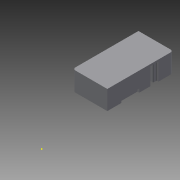
# Autodesk Inventor part: Positive CAp
Saved by Autodesk Inventor 2015 (Build 190159000, 159)
## iProperties
Created: 2015-01-23
Part Number: Positive CAp
Material: Generic
Document SubType Name: Modeling
Designer: pltwe4
Density: 1 g/cm^3
Appearance: Default
Author: pltwe4
Autodesk Inventor part; units mm, degrees
ref_plane "YZ Plane" through (0, 0, 0) normal (1, 0, 0) x (0, 1, 0)
ref_plane "XZ Plane" through (0, 0, 0) normal (0, 1, 0) x (-1, 0, 0)
ref_plane "XY Plane" through (0, 0, 0) normal (0, 0, 1) x (1, 0, 0)
sketch "Sketch1" plane through (0, 0, 0) normal (0, 1, 0) x (-1, 0, 0)
  line L0 (0, 0) -> (24.5364, 0)
  line L1 (24.5364, 0) -> (24.5364, -46.5582)
  line L2 (24.5364, -46.5582) -> (0, -46.5582)
  line L3 (0, -46.5582) -> (0, 0)
  dimension "d0" = 46.5582
  dimension "d1" = 24.5364
  constraints: 8 end point, 2 parallel, 1 horizontal, 1 perpendicular
  measures "d0" distance of L0.end L1.end
  measures "d1" distance of L1.end L2.end
extrude "Extrusion1" add sketch "Sketch1" along normal blind 13.5382
sketch "Sketch2" plane through (0, 0, 0) normal (0, -1, 0) x (1, 0, 0)
  point P0 (0, 0)
fillet "Fillet1" radius 1.905 1 edges at (-24.5364, 6.7691, -46.5582)
fillet "Fillet2" radius 1.905 1 edges at (0, 6.7691, 0)
sketch "Sketch3" plane through (0, 0, 0) normal (0, -1, 0) x (1, 0, 0)
  line L0 (-1.905, 0) -> (-24.5364, 0) projected
  arc A0 (0, -1.905) -> (-1.905, 0) centre (-1.905, -1.905) ccw projected
  line L1 (0, -46.5582) -> (0, -1.905) projected
  line L2 (-22.6314, -46.5582) -> (0, -46.5582) projected
  arc A1 (-24.5364, -44.6532) -> (-22.6314, -46.5582) centre (-22.6314, -44.6532) ccw projected
  line L3 (-24.5364, 0) -> (-24.5364, -44.6532) projected
  line L4 (-2.54, -2.54) -> (-21.9964, -2.54)
  line L5 (-21.9964, -44.0182) -> (-2.54, -44.0182)
  line L6 (0, -12.9032) -> (-5.08, -12.9032)
  line L7 (-5.08, -16.0782) -> (0, -16.0782)
  line L8 (-2.54, -44.0182) -> (-2.54, -18.6182)
  line L9 (-2.54, -10.3632) -> (-2.54, -2.54)
  line L10 (-5.08, -12.9032) -> (-5.08, -10.3632)
  line L11 (-5.08, -10.3632) -> (-2.54, -10.3632)
  line L12 (-5.08, -16.0782) -> (-5.08, -18.6182)
  line L13 (-5.08, -18.6182) -> (-2.54, -18.6182)
  line L14 (-21.9964, -10.3632) -> (-18.4404, -10.3632)
  line L15 (-18.4404, -10.3632) -> (-18.4404, -18.6182)
  line L16 (-18.4404, -18.6182) -> (-21.9964, -18.6182)
  line L17 (-21.9964, -2.54) -> (-21.9964, -10.3632)
  line L18 (-21.9964, -18.6182) -> (-21.9964, -44.0182)
  line L19 (0, -14.4907) -> (-5.2569, -14.4907) construction
  line L20 (-5.08, -11.6332) -> (-18.4404, -11.6332)
  line L21 (-5.08, -17.3482) -> (-18.4404, -17.3482)
  point P0 (0, 0)
  dimension "d7" = 2.54
  dimension "d9" = 2.54
  dimension "d11" = 3.175
  dimension "d13" = 5.08
  dimension "d14" = 2.54
  dimension "d15" = 2.54
  dimension "d16" = 2.54
  dimension "d17" = 2.54
  dimension "d20" = 2.54
  dimension "d21" = 6.096
  dimension "d22" = 2.54
  dimension "d37" = 32.0675
  constraints: 36 end point, 9 perpendicular, 7 parallel, 5 point on line, 4 horizontal, 2 collinear, 2 midpoint, 2 vertical, 1 other
  measures "d7" distance between parallel lines of L0 L4
  measures "d9" distance between parallel lines of L2 L5
  measures "d11" distance between parallel lines of L6 L7
  measures "d13" distance between parallel lines of L1 L10
  measures "d14" distance of L7.start L12.end
  measures "d15" distance of L6.end L10.end
  measures "d16" distance between parallel lines of L1 L8
  measures "d17" distance between parallel lines of L1 L9
  measures "d20" distance between parallel lines of L3 L18
  measures "d21" distance between parallel lines of L3 L15
  measures "d22" distance between parallel lines of L3 L17
  measures "d37" distance between parallel lines of L2 L19
extrude "Extrusion2" cut sketch "Sketch3" against normal blind 12.2682 contours L1 L7 L12 L21 L15 L20 L10 L6 | L20 L15 L14 L17 L4 L9 L11 L10 | L12 L13 L8 L5 L18 L16 L15 L21
sketch "Sketch4" plane through (0, 12.2682, 0) normal (0, -1, 0) x (1, 0, 0)
  line L0 (-4.3434, -23.6982) -> (-17.0434, -23.6982)
  line L1 (-17.0434, -23.6982) -> (-17.0434, -35.1282)
  line L2 (-17.0434, -35.1282) -> (-4.3434, -35.1282)
  line L3 (-4.3434, -35.1282) -> (-4.3434, -23.6982)
  line L4 (-2.54, -44.0182) -> (-21.9964, -44.0182) projected
  line L5 (-2.54, -18.6182) -> (-2.54, -44.0182) projected
  line L6 (-10.6934, -23.6982) -> (-10.6934, -35.1282) construction
  line L7 (-24.5364, 0) -> (-24.5364, -44.6532) construction
  line L8 (-22.6314, -46.5582) -> (0, -46.5582) construction
  point P0 (0, 0)
  dimension "d23" = 13.843
  dimension "d24" = 12.7
  dimension "d25" = 11.43
  dimension "d26" = 22.86
  constraints: 10 end point, 2 midpoint, 2 parallel, 1 horizontal, 1 perpendicular
  measures "d23" distance between parallel lines of L7 L6
  measures "d24" distance between parallel lines of L1 L3
  measures "d25" distance between parallel lines of L0 L2
  measures "d26" distance between parallel lines of L8 L0
extrude "Extrusion3" add sketch "Sketch4" along normal up to surface (12.2682 mm away)
sketch "Sketch5" plane through (-4.3434, 12.2682, -35.1282) normal (0, 0, -1) x (-1, 0, 0)
  line L0 (0, 0) -> (0, -12.2682) projected
  line L1 (12.7, 0) -> (12.7, -12.2682) projected
  line L2 (12.7, -12.2682) -> (0, -12.2682) projected
  arc A0 (8.2396, -6.5778) -> (4.4604, -6.5778) centre (6.35, -5.1816) ccw
  line L3 (6.35, -12.2682) -> (6.35, 0) construction
  line L4 (17.653, 0) -> (-1.8034, 0) construction
  line L5 (8.2396, -6.5778) -> (8.4707, -7.62)
  line L6 (8.4707, -7.62) -> (11.0107, -7.62)
  line L7 (11.0107, -7.62) -> (12.7, 0)
  line L8 (4.4604, -6.5778) -> (4.2293, -7.62)
  line L9 (4.2293, -7.62) -> (1.6893, -7.62)
  line L10 (1.6893, -7.62) -> (0, 0)
  point P0 (-4.3434, -12.2682)
  dimension "d29" = 7.0866
  dimension "d30" = 4.699
  dimension "d32" = 7.62
  dimension "d33" = 2.54
  dimension "d36" = 25
  constraints: 14 end point, 2 horizontal, 2 point on circle, 2 point on line, 1 centre point, 1 equal length, 1 midpoint, 1 parallel, 1 vertical, 2 other
  measures "d29" distance from line of L2 A0.centre
  measures "d30" diameter of A0
  measures "d32" distance between parallel lines of L4 L6
  measures "d33" distance of L5.end L6.end
  measures "d36" angle of L5 L8
extrude "Extrusion4" cut sketch "Sketch5" against normal up to surface (11.43 mm away)
sketch "Sketch6" plane through (0, 12.2682, 0) normal (0, -1, 0) x (1, 0, 0)
  line L0 (-5.08, -10.3632) -> (-5.08, -12.9032) projected
  line L1 (-5.08, -16.0782) -> (-5.08, -18.6182) projected
  line L2 (-18.4404, -18.6182) -> (-18.4404, -10.3632) projected
  line L3 (0, -12.9032) -> (0, -16.0782) projected
  line L4 (0, -16.0782) -> (-5.08, -16.0782) projected
  line L5 (-5.08, -12.9032) -> (0, -12.9032) projected
  line L6 (-5.08, -10.3632) -> (-18.4404, -10.3632)
  line L7 (-18.4404, -18.6182) -> (-5.08, -18.6182)
  line L8 (-1.27, -12.9032) -> (-1.27, -16.0782)
  point P0 (0, 0)
  dimension "d46" = 1.27
  constraints: 6 end point, 2 point on line, 1 horizontal, 1 parallel, 1 perpendicular
  measures "d46" distance between parallel lines of L8 L3
extrude "Extrusion5" cut sketch "Sketch6" against normal blind 0.635
sketch "Sketch7" plane through (0, 0, 0) normal (0, -1, 0) x (1, 0, 0)
  line L0 (0, -12.9032) -> (0, -1.905) projected
  line L1 (0, -1.905) -> (0, -46.5582) projected
  line L2 (0, -10.3632) -> (-0.635, -10.3632)
  line L3 (-1.27, -10.9982) -> (-1.27, -12.2682)
  arc A0 (-0.635, -10.3632) -> (-1.27, -10.9982) centre (-0.635, -10.9982) ccw
  line L4 (-1.905, -12.9032) -> (-5.08, -12.9032)
  line L5 (-5.08, -10.3632) -> (-5.08, -12.9032) projected
  arc A1 (-1.905, -12.9032) -> (-1.27, -12.2682) centre (-1.905, -12.2682) ccw
  line L6 (0, -10.3632) -> (0, -12.9032)
  line L7 (0, -12.9032) -> (-1.905, -12.9032)
  line L8 (-5.08, -12.9032) -> (0, -12.9032) projected
  point P0 (0, 0)
  point P1 (-1.27, -10.3632)
  point P2 (-1.27, -12.9032)
  dimension "d40" = 1.27
  dimension "d41" = 2.54
  dimension "d42" = 0.635
  dimension "d43" = 0.635
  constraints: 10 end point, 5 point on line, 5 tangent, 4 point on circle, 2 centre point, 2 collinear, 2 perpendicular, 1 parallel
  measures "d40" distance of L2.start point (-1.27, -10.363)
  measures "d41" distance of point (-1.27, -10.363) point (-1.27, -12.903)
  measures "d42" radius of A0
  measures "d43" radius of A1
extrude "Extrusion7" add sketch "Sketch6" against normal blind 0.635 contours L5 L3 L4 L8
extrude "Extrusion8" cut sketch "Sketch7" against normal up to surface (12.2682 mm away)
sketch "Sketch8" plane through (0, 0, -46.5582) normal (1, 0, 0) x (0, 0, -1)
  line L0 (-36.195, 0) -> (-36.195, 12.2682) projected
  line L1 (-30.48, 12.2682) -> (-36.195, 12.2682) projected
  line L2 (-30.48, 12.2682) -> (-30.48, 0) projected
  line L3 (0, 0) -> (-30.48, 0) projected
  line L4 (0, 0) -> (0, 13.5382) projected
  line L5 (-44.6532, 13.5382) -> (0, 13.5382) projected
  line L6 (-44.6532, 0) -> (-44.6532, 13.5382) projected
  line L7 (-36.195, 0) -> (-44.6532, 0) projected
  line L8 (-22.5397, 0) -> (-22.5397, 2.54)
  line L9 (-22.5397, 2.54) -> (-9.8397, 2.54)
  line L10 (-9.8397, 2.54) -> (-9.8397, 0)
  point P0 (-46.5582, 0)
  dimension "d51" = 2.54
  dimension "d52" = 12.7
  constraints: 6 end point, 2 perpendicular, 2 point on line, 1 vertical
  measures "d51" distance of L9.end L10.end
  measures "d52" distance of L8.end L9.end
extrude "Extrusion9" cut sketch "Sketch8" against normal blind 1.27 contours L8 L9 L10 L3
sketch "Sketch9" plane through (-4.3434, 12.2682, -35.1282) normal (0, 0, -1) x (-1, 0, 0)
  line L0 (12.7, 0) -> (11.0107, -7.62) projected
  line L1 (11.0107, -7.62) -> (8.4707, -7.62) projected
  line L2 (8.4707, -7.62) -> (8.2396, -6.5778) projected
  arc A0 (8.2396, -6.5778) -> (4.4604, -6.5778) centre (6.35, -5.1816) ccw projected
  line L3 (4.4604, -6.5778) -> (4.2293, -7.62) projected
  line L4 (4.2293, -7.62) -> (1.6893, -7.62) projected
  line L5 (1.6893, -7.62) -> (0, 0) projected
  line L6 (12.7, 0) -> (0, 0) projected
  line L7 (1.6893, -7.62) -> (11.0107, -7.62)
  line L8 (4.2293, -7.62) -> (1.6893, -7.62) projected
  point P0 (-4.3434, -12.2682)
  constraints: 2 end point, 1 collinear
extrude "Extrusion10" add sketch "Sketch9" along normal blind 2.54
mirror "Mirror1" about plane through (0, 0, -46.5582) normal (0, 0, -1) remove original yes
equation "\"d27\" = d2"
equation "\"d34\" = d2"
equation "\"d2\" = 13.5382"
body "Solid1"
